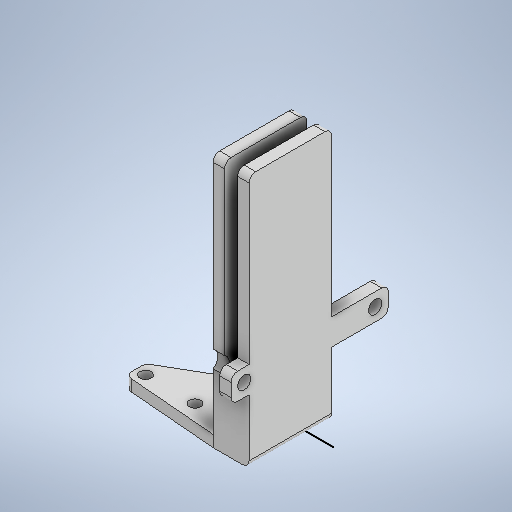
# Autodesk Inventor part: nasilnikprzod2_new
Saved by Autodesk Inventor 2025.2 (Build 292293000, 293)
## iProperties
Created: 2025-09-01
Part Number: nasilnikprzod2_new
Material: Ogólny
Document SubType Name: Modeling
Designer: janla
Density: 1 g/cm^3
Appearance: Domyślna
Author: janla
Autodesk Inventor part; units mm, degrees
ref_plane "YZ Plane" through (0, 0, 0) normal (1, 0, 0) x (0, 1, 0)
ref_plane "XZ Plane" through (0, 0, 0) normal (0, 1, 0) x (-1, 0, 0)
ref_plane "XY Plane" through (0, 0, 0) normal (0, 0, 1) x (1, 0, 0)
sketch "Szkic1" plane through (0, 0, 0) normal (0, 1, 0) x (-1, 0, 0)
  circle A0 centre (0, 0) radius 18.5
  circle A1 centre (0, 0) radius 15.125
  line L0 (15.125, 0) -> (7.5625, -13.0986)
  line L1 (7.5625, -13.0986) -> (-7.5625, -13.0986)
  line L2 (-7.5625, -13.0986) -> (-15.125, 0)
  line L3 (-15.125, 0) -> (-7.5625, 13.0986)
  line L4 (-7.5625, 13.0986) -> (7.5625, 13.0986)
  line L5 (7.5625, 13.0986) -> (15.125, 0)
  circle A2 centre (-15.125, 0) radius 1.75
  circle A3 centre (-7.5625, -13.0986) radius 1.75
  circle A4 centre (7.5625, -13.0986) radius 1.75
  line L6 (-18.5, 0) -> (-29.5, 0)
  line L7 (-29.5, 0) -> (-29.5, -18.5)
  line L8 (-29.5, -18.5) -> (-18.5, -18.5)
  line L9 (-18.5, -18.5) -> (-18.5, 0)
  line L10 (-29.5, -18.5) -> (-26, -18.5)
  line L11 (-26, -18.5) -> (-26, 0)
  line L12 (-26, 0) -> (-29.5, 0)
  line L13 (-29.5, 0) -> (-29.5, -18.5)
  line L14 (-26, -18.5) -> (-22, -18.5)
  line L15 (-22, -18.5) -> (-22, 0)
  line L16 (-22, 0) -> (-26, 0)
  line L17 (-26, 0) -> (-26, -18.5)
  line L18 (-18.5, 0) -> (-29.5, 0)
  line L19 (-29.5, 0) -> (-29.5, 15)
  line L20 (7.5625, -13.0986) -> (-18.5, -13.0986)
  line L21 (-18.5, -13.0986) -> (-18.5, -16.0986)
  line L22 (-18.5, -16.0986) -> (7.5625, -16.0986)
  line L23 (7.5625, -16.0986) -> (7.5625, -13.0986)
  line L24 (7.5625, -10.0986) -> (7.5625, -16.0986)
  line L25 (7.5625, -10.0986) -> (-18.5, -10.0986)
  line L26 (-18.5, -10.0986) -> (-18.5, -13.0986)
  line L27 (-18.5, -13.0986) -> (7.5625, -13.0986)
  line L28 (7.5625, -13.0986) -> (7.5625, -10.0986)
  line L29 (7.5625, -10.0986) -> (10.5625, -10.0986)
  line L30 (10.5625, -10.0986) -> (10.5625, -16.0986)
  line L31 (10.5625, -16.0986) -> (7.5625, -16.0986)
  line L32 (7.5625, -16.0986) -> (7.5625, -10.0986)
  line L33 (10.5625, -10.0986) -> (-18.5, 6.6806)
  line L34 (-18.5, -18.5) -> (10.5625, -16.0986)
  line L35 (-18.5, 6.6806) -> (-29.5, 13.0315)
  line L36 (-29.5, 0) -> (-18.5, 0)
  line L37 (-18.5, 0) -> (-18.5, 6.6806)
  line L38 (-18.5, 6.6806) -> (-29.5, 6.6806)
  line L39 (-29.5, 6.6806) -> (-29.5, 0)
  point P0 (-9.3125, -13.0986)
  point P1 (-5.8125, -13.0986)
  point P2 (5.8125, -13.0986)
  point P3 (7.5625, -14.8486)
  dimension "d0" = 37
  dimension "d1" = 30.25
  dimension "d2" = 3.5
  dimension "d3" = 3.5
  dimension "d4" = 3.5
  dimension "d5" = 11
  dimension "d6" = 3.5
  dimension "d7" = 4
  dimension "d9" = 3
  dimension "d10" = 3
  dimension "d12" = 3
  dimension "d13" = 30
  constraints: 80 end point, 14 parallel, 8 horizontal, 8 perpendicular, 6 coincident, 4 point on line, 3 centre point, 2 horizontal alignment, 17 other
  measures "d2" diameter of A2
  measures "d3" diameter of A3
  measures "d4" diameter of A4
  measures "d5" distance of L8.end L7.end
  measures "d6" distance of L12.end L11.end
  measures "d7" distance of L16.end L15.end
  measures "d9" distance between parallel lines of L22 L1
  measures "d10" distance between parallel lines of L25 L1
  measures "d12" distance of L30.end L31.end
  measures "d13" angle of L33 L25
extrude "Wyciągnięcie proste1" add sketch "Szkic1" along normal blind 3.5 contours L33 A1 A2 L25 A0 | A0 L37 L33 | L30 L31 A0 | A0 L31 L23 A4 A1 L30 | L9 L8 L15 L6 | A0 L25 L9 | L6 L19 L38 L37 | L33 L3 A2 A1 | L31 L34 A0 | A0 L34 L22 L31 | A1 A4 L0 L29 L30 | L25 A1 A3 L20 A0 | A0 L20 L9 L25 | L15 L8 L11 L6 | L33 L0 L29 L25 L2 A2 L3 | L22 A0 L20 A3 A1 A4 L23 | L29 L0 L33 | A0 L22 L9 L20 | L25 L2 A3 A1 | A1 A2 L2 L25 | L11 L8 L7 L6 | L34 L9 L22 A0 | A4 L24 L29 L0 | L25 L24 A4 L1 A3 L2 | A1 A3 L1 A4
sketch "Szkic2" plane through (0, 3.5, 0) normal (0, 1, 0) x (1, 0, 0)
  line L0 (18.5, -6.6806) -> (29.5, -6.6806) projected
  line L1 (18.5, 18.5) -> (-10.5625, 16.0986) projected
  line L2 (29.5, -6.6806) -> (18.5, -6.6806)
  line L3 (18.5, -6.6806) -> (18.5, 18.5)
  line L4 (18.5, 18.5) -> (29.5, 18.5)
  line L5 (29.5, 18.5) -> (29.5, -6.6806)
  point P0 (0, 0)
  constraints: 8 end point, 2 parallel, 1 horizontal, 1 perpendicular
extrude "Wyciągnięcie proste2" add sketch "Szkic2" along normal blind 74
sketch "Szkic3" plane through (0, 77.5, 0) normal (0, 1, 0) x (1, 0, 0)
  line L0 (18.5, -6.6806) -> (29.5, -6.6806) projected
  line L1 (29.5, 18.5) -> (18.5, 18.5) projected
  line L2 (26, -6.6806) -> (22, -6.6806)
  line L3 (22, -6.6806) -> (22, 18.5)
  line L4 (22, 18.5) -> (26, 18.5)
  line L5 (26, 18.5) -> (26, -6.6806)
  line L6 (18.5, 18.5) -> (18.5, -6.6806) projected
  point P0 (0, 0)
  dimension "d21" = 4
  dimension "d22" = 3.5
  constraints: 8 end point, 2 parallel, 2 point on line, 1 horizontal, 1 perpendicular
  measures "d21" distance of L3.end L4.end
  measures "d22" distance between parallel lines of L6 L3
extrude "Wyciągnięcie proste3" cut sketch "Szkic3" against normal blind 60 contours L3 L1 L5 L0
sketch "Szkic4" plane through (0, 17.5, 0) normal (0, 1, 0) x (1, 0, 0)
  line L0 (26, 18.5) -> (26, -6.6806) projected
  line L1 (22, -6.6806) -> (22, 18.5) projected
  line L2 (22, 0) -> (22, 11.8194)
  line L3 (26, 11.8194) -> (26, 0)
  line L4 (26, -6.6806) -> (22, -6.6806) projected
  line L5 (22, 18.5) -> (26, 18.5) projected
  line L6 (22, 14.5) -> (26, 14.5)
  line L7 (26, 14.5) -> (26, -2.6806)
  line L8 (26, -2.6806) -> (22, -2.6806)
  line L9 (22, -2.6806) -> (22, 14.5)
  point P0 (0, 0)
  dimension "d29" = 4
  dimension "d30" = 4
  constraints: 12 end point, 4 point on line, 3 parallel, 1 horizontal, 1 perpendicular
  measures "d29" distance between parallel lines of L5 L6
  measures "d30" distance between parallel lines of L4 L8
extrude "Wyciągnięcie proste4" cut sketch "Szkic4" against normal blind 60 contours L0 L8 L1 L6
sketch "Szkic8" plane through (29.5, 0, 6.6806) normal (1, 0, 0) x (0, 0, -1)
  line L0 (-17, 23.5) -> (25.1806, 23.5)
  line L1 (25.1806, 0) -> (25.1806, 77.5) projected
  line L2 (6.6806, 0) -> (6.6806, 23.5)
  line L3 (6.6806, 18.5) -> (30.6806, 18.5)
  line L4 (30.6806, 18.5) -> (30.6806, 28.5)
  line L5 (30.6806, 28.5) -> (6.6806, 28.5)
  line L6 (6.6806, 28.5) -> (6.6806, 18.5)
  line L7 (6.6806, 18.5) -> (-17.3194, 18.5)
  line L8 (-17.3194, 18.5) -> (-17.3194, 28.5)
  line L9 (-17.3194, 28.5) -> (6.6806, 28.5)
  line L10 (6.6806, 28.5) -> (6.6806, 18.5)
  line L11 (30.6806, 23.5) -> (-17.3194, 23.5)
  line L12 (30.6806, 19.5) -> (-17.3194, 19.5)
  line L13 (-17.3194, 19.5) -> (-17.3194, 27.5)
  line L14 (-17.3194, 27.5) -> (30.6806, 27.5)
  line L15 (30.6806, 27.5) -> (30.6806, 19.5)
  point P0 (25.1806, 28.5)
  point P1 (25.1806, 18.5)
  point P2 (25.1806, 27.5)
  point P3 (25.1806, 19.5)
  point P4 (6.6806, 27.5)
  point P5 (6.6806, 19.5)
  dimension "d39" = 24
  dimension "d40" = 24
  dimension "d47" = 1
  dimension "d48" = 1
  constraints: 30 end point, 6 parallel, 6 point on line, 4 horizontal, 4 perpendicular, 2 midpoint
  measures "d39" distance of L5.end L4.end
  measures "d40" distance of L8.end L9.end
  measures "d47" distance between parallel lines of L12 L7
  measures "d48" distance between parallel lines of L14 L9
extrude "Wyciągnięcie proste6" add sketch "Szkic8" against normal blind 3.5 contours L11 L8 L14 L6 L0 | L0 L2 L12 L8 L11 | L11 L4 L12 L1 | L1 L14 L4 L11
sketch "Szkic9" plane through (26, 77.5, -18.5) normal (-1, 0, 0) x (0, 0, 1)
  line L0 (42.5, -58) -> (42.5, -50) projected
  line L1 (42.5, -54) -> (38.5, -54)
  circle A0 centre (38.5, -54) radius 2
  line L2 (-5.5, -50) -> (-5.5, -58) projected
  line L3 (-5.5, -54) -> (-1.5, -54)
  circle A1 centre (-1.5, -54) radius 2
  point P0 (18.5, -77.5)
  point P1 (42.5, -59)
  point P2 (42.5, -49)
  point P3 (-5.5, -49)
  point P4 (-5.5, -59)
  dimension "d43" = 4
  dimension "d44" = 4
  dimension "d45" = 4
  dimension "d46" = 4
  constraints: 4 end point, 2 centre point, 2 coincident, 2 horizontal, 2 midpoint
  measures "d43" distance of L1.start L1.end
  measures "d44" diameter of A0
  measures "d45" distance of L3.start L3.end
  measures "d46" diameter of A1
extrude "Wyciągnięcie proste7" cut sketch "Szkic9" along normal mid plane 50
fillet "Zaokrąglenie3" radius 2 11 edges at (-10.5625, 1.75, -16.0986) (-10.5625, 1.75, -10.0986) (29.5, 0, -5.9097) (27.75, 19.5, 24) (27.75, 27.5, 24) (27.75, 19.5, -24) (27.75, 27.5, -24) (27.75, 77.5, -18.5) (27.75, 77.5, 6.6806) (20.25, 77.5, 6.6806) (20.25, 77.5, -18.5)
sketch "Szkic10" plane through (18.5, 3.5, -18.5) normal (-1, 0, 0) x (0, 0, 1)
  circle A0 centre (-1.5, 20) radius 2 projected
  circle A1 centre (-1.5, 20) radius 3
  point P0 (18.5, -3.5)
  dimension "d52" = 6
  constraints: 1 centre point, 1 coincident
  measures "d52" diameter of A1
extrude "Wyciągnięcie proste8" cut sketch "Szkic10" against normal blind 4 contours A0 | A1
sketch "Szkic11" plane through (0, 0, 0) normal (0, -1, 0) x (1, 0, 0)
  line L0 (0, 0) -> (36.7691, 0)
  constraints: 2 end point, 1 horizontal
mirror "Odbij1" about plane through (0, 0, 0) normal (0, 0, 1) remove original yes
